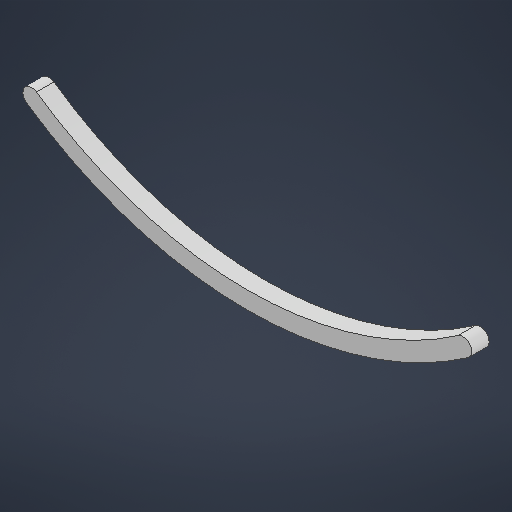
# Autodesk Inventor part: Saddle
Saved by Autodesk Inventor 2026 (Build 300175000, 175)
## iProperties
Created: 2025-10-31
Part Number: Saddle
Material: Generic
Document SubType Name: Modeling
Designer: Brandon Portillo
Density: 1 g/cm^3
Appearance: Default
Author: Brandon Portillo
Autodesk Inventor part; units mm, degrees
ref_plane "YZ Plane" through (0, 0, 0) normal (1, 0, 0) x (0, 1, 0)
ref_plane "XZ Plane" through (0, 0, 0) normal (0, 1, 0) x (-1, 0, 0)
ref_plane "XY Plane" through (0, 0, 0) normal (0, 0, 1) x (1, 0, 0)
sketch "Sketch1" plane through (0, 0, 0) normal (0, 0, 1) x (1, 0, 0)
  arc A0 (0, -2125) -> (1212.8796, -1744.8633) centre (0, 0) ccw
  arc A1 (0, -2225) -> (1269.9563, -1826.9745) centre (0, 0) ccw
  line L0 (0, -2125) -> (0, -1744.8633)
  arc A2 (1269.9563, -1826.9745) -> (1212.8796, -1744.8633) centre (1241.418, -1785.9189) ccw
  line L1 (0, -2225) -> (0, -2125)
  arc A3 (-1212.8796, -1744.8633) -> (0, -2125) centre (0, 0) ccw
  arc A4 (-1269.9563, -1826.9745) -> (0, -2225) centre (0, 0) ccw
  arc A5 (-1212.8796, -1744.8633) -> (-1269.9563, -1826.9745) centre (-1241.418, -1785.9189) ccw
  dimension "d0" = 4250
  dimension "d1" = 4450
  constraints: 12 point on circle, 6 centre point, 4 end point, 3 coincident, 3 symmetric about line, 2 vertical, 1 tangent, 3 other
  measures "d0" diameter of A0
  measures "d1" diameter of A1
extrude "Extrusion1" add sketch "Sketch1" along normal blind 100
body "Solid1"
